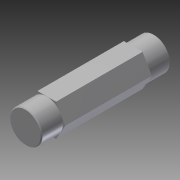
# Autodesk Inventor part: DBK_SmallHexShaft_am-0152
Saved by Autodesk Inventor 2014 (Build 180170000, 170)
## iProperties
Category: Drive Base Kit
Company: Autodesk Inc.
Created: 2012-12-19
Part Number: DBK_SmallHexShaft_am-0152
Material: Steel
Document SubType Name: Modeling
Designer: Autodesk Inc.
Density: 7.83431 g/cm^3
Catalog Web Link: http://www.andymark.com/product-p/am-0152.htm
Vendor: AndyMark Inc.
Mass: 22.6796 g
Surface Area: 13.656 cm^2
Volume: 2.89491 cm^3
Appearance: Steel
Author: Autodesk Inc.
Autodesk Inventor part; units mm, degrees
ref_plane "YZ Plane" through (0, 0, 0) normal (1, 0, 0) x (0, 1, 0)
ref_plane "XZ Plane" through (0, 0, 0) normal (0, 1, 0) x (-1, 0, 0)
sketch "Sketch1" plane through (0, 0, 0) normal (0, 0, 1) x (1, 0, 0)
  line L0 (2.7496, 4.7625) -> (5.4993, 0)
  line L1 (5.4993, 0) -> (2.7496, -4.7625)
  line L2 (2.7496, -4.7625) -> (-2.7496, -4.7625)
  line L3 (-2.7496, -4.7625) -> (-5.4993, 0)
  line L4 (-5.4993, 0) -> (-2.7496, 4.7625)
  line L5 (-2.7496, 4.7625) -> (2.7496, 4.7625)
  point P0 (0, 0)
  point P1 (0, 0)
  dimension "d0" = 9.525
  constraints: 12 end point, 1 coincident, 1 horizontal, 13 other
  measures "d0" distance between parallel lines of L2 L5
extrude "Extrusion1" add sketch "Sketch1" against normal blind 38.1
sketch "Sketch2" plane through (0, 0, 0) normal (0, 0, 1) x (1, 0, 0)
  line L0 (2.7496, 4.7625) -> (5.4993, 0) projected
  line L1 (-2.7496, 4.7625) -> (2.7496, 4.7625) projected
  line L2 (-5.4993, 0) -> (-2.7496, 4.7625) projected
  line L3 (-2.7496, -4.7625) -> (-5.4993, 0) projected
  line L4 (2.7496, -4.7625) -> (-2.7496, -4.7625) projected
  line L5 (5.4993, 0) -> (2.7496, -4.7625) projected
  circle A0 centre (0, 0) radius 4.7498
  dimension "d3" = 9.4996
  constraints: 1 centre point, 1 coincident
  measures "d3" diameter of A0
extrude "Extrusion2" cut sketch "Sketch2" against normal blind 6.2865
ref_plane "Work Plane1" through (0, 0, -19.05) normal (0, 0, 1) x (1, 0, 0)
mirror "Mirror1" about plane through (0, 0, -19.05) normal (0, 0, 1) of "Extrusion2"
chamfer "Chamfer1" distance 0.254 angle 45 2 edges at (-4.7498, 0, 0) (-4.7498, 0, -38.1)
body "Solid1"
